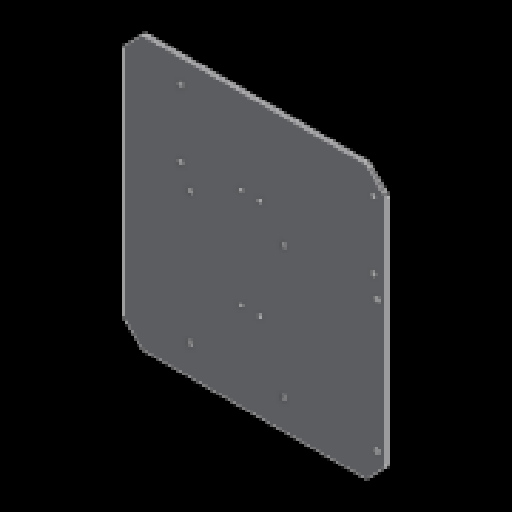
# Autodesk Inventor part: ChestTopPanel
Saved by Autodesk Inventor 2025.2 (Build 292293000, 293)
## iProperties
Created: 2025-10-05
Part Number: ChestTopPanel
Material: Generic
Document SubType Name: Sheet Metal
Designer: valer
Density: 1 g/cm^3
Sheet Metal Rule: Default
Appearance: Default
Author: valer
Autodesk Inventor part; units mm, degrees
ref_plane "YZ Plane" through (0, 0, 0) normal (1, 0, 0) x (0, 1, 0)
ref_plane "XZ Plane" through (0, 0, 0) normal (0, 1, 0) x (-1, 0, 0)
ref_plane "XY Plane" through (0, 0, 0) normal (0, 0, 1) x (1, 0, 0)
sketch "Base" plane through (0, 0, 0) normal (0, 0, 1) x (1, 0, 0)
  line L0 (370.5814, -184.5855) -> (20.5814, -184.5855)
  line L1 (20.5814, -184.5855) -> (20.5814, 180.4145)
  line L2 (20.5814, 180.4145) -> (370.5814, 180.4145)
  line L3 (370.5814, 180.4145) -> (370.5814, -184.5855)
  point P0 (0, 0)
  dimension "d1" = 365
  dimension "d3" = 350
  measures "d1" distance of L2.end L0.start
  measures "d3" distance of L0.start L0.end
extrude "Plate1" add sketch "Base" along normal blind 5
chamfer "BaseChamfersFeature" distance 25 angle 45 4 edges at (20.5814, 180.4145, 2.5) (370.5814, 180.4145, 2.5) (370.5814, -184.5855, 2.5) (20.5814, -184.5855, 2.5)
fillet "BaseFilletsFeature" radius 8 8 edges at (20.5814, 155.4145, 2.5) (45.5814, 180.4145, 2.5) (20.5814, -159.5855, 2.5) (45.5814, -184.5855, 2.5) (345.5814, 180.4145, 2.5) (370.5814, 155.4145, 2.5) (370.5814, -159.5855, 2.5) (345.5814, -184.5855, 2.5)
sketch "PowerSupplyBracketMountHoles" plane through (0, 0, 0) normal (0, 0, -1) x (-1, 0, 0)
  circle A0 centre (-360.5814, 31.4145) radius 3 projected
  circle A1 centre (-235.5814, 31.4145) radius 3 projected
  circle A2 centre (-110.5814, 31.4145) radius 3 projected
  circle A3 centre (-360.5814, -144.5855) radius 3 projected
  circle A4 centre (-235.5814, -144.5855) radius 3 projected
  circle A5 centre (-110.5814, -144.5855) radius 3 projected
  point P0 (0, 0)
extrude "PowerSupplyBracketMountHolesFeature" cut sketch "PowerSupplyBracketMountHoles" against normal blind 5
sketch "ChargerMountHoles" plane through (0, 0, 0) normal (0, 0, -1) x (-1, 0, 0)
  line L0 (-338.5814, 164.0145) -> (-338.5814, 43.4145) construction
  line L1 (-338.5814, 43.4145) -> (-358.8814, 43.4145) construction
  arc A0 (-364.5814, 49.1145) -> (-358.8814, 43.4145) centre (-358.8814, 49.1145) ccw construction
  line L2 (-364.5814, 49.1145) -> (-364.5814, 55.9145) construction
  line L3 (-364.5814, 55.9145) -> (-355.4314, 55.9145) construction
  arc A1 (-355.4314, 55.9145) -> (-355.4314, 61.6145) centre (-355.4314, 58.7645) ccw construction
  line L4 (-355.4314, 61.6145) -> (-364.5814, 61.6145) construction
  line L5 (-364.5814, 61.6145) -> (-364.5814, 145.8145) construction
  line L6 (-364.5814, 145.8145) -> (-355.4314, 145.8145) construction
  arc A2 (-355.4314, 145.8145) -> (-355.4314, 151.5145) centre (-355.4314, 148.6645) ccw construction
  line L7 (-355.4314, 151.5145) -> (-364.5814, 151.5145) construction
  line L8 (-364.5814, 151.5145) -> (-364.5814, 158.3145) construction
  arc A3 (-358.8814, 164.0145) -> (-364.5814, 158.3145) centre (-358.8814, 158.3145) ccw construction
  line L9 (-358.8814, 164.0145) -> (-338.5814, 164.0145) construction
  line L10 (-114.5814, 43.4145) -> (-114.5814, 164.0145) construction
  line L11 (-114.5814, 164.0145) -> (-94.2814, 164.0145) construction
  arc A4 (-88.5814, 158.3145) -> (-94.2814, 164.0145) centre (-94.2814, 158.3145) ccw construction
  line L12 (-88.5814, 158.3145) -> (-88.5814, 151.5145) construction
  line L13 (-88.5814, 151.5145) -> (-97.7314, 151.5145) construction
  arc A5 (-97.7314, 151.5145) -> (-97.7314, 145.8145) centre (-97.7314, 148.6645) ccw construction
  line L14 (-97.7314, 145.8145) -> (-88.5814, 145.8145) construction
  line L15 (-88.5814, 145.8145) -> (-88.5814, 61.6145) construction
  line L16 (-88.5814, 61.6145) -> (-97.7314, 61.6145) construction
  arc A6 (-97.7314, 61.6145) -> (-97.7314, 55.9145) centre (-97.7314, 58.7645) ccw construction
  line L17 (-97.7314, 55.9145) -> (-88.5814, 55.9145) construction
  line L18 (-88.5814, 55.9145) -> (-88.5814, 49.1145) construction
  arc A7 (-94.2814, 43.4145) -> (-88.5814, 49.1145) centre (-94.2814, 49.1145) ccw construction
  line L19 (-94.2814, 43.4145) -> (-114.5814, 43.4145) construction
  circle A8 centre (-97.7314, 58.7645) radius 2.5
  circle A9 centre (-97.7314, 148.6645) radius 2.5
  circle A10 centre (-355.4314, 58.7645) radius 2.5
  circle A11 centre (-355.4314, 148.6645) radius 2.5
  point P0 (0, 0)
  dimension "d14" = 5
  constraints: 4 centre point, 4 coincident, 3 equal radius
  measures "d14" diameter of A8
extrude "ChargerMountHolesFeature" cut sketch "ChargerMountHoles" against normal blind 5
sketch "USBHubMountHoles" plane through (0, 0, 0) normal (0, 0, -1) x (-1, 0, 0)
  circle A0 centre (-178.2994, 66.75) radius 2.25 construction
  circle A1 centre (-203.2994, 66.75) radius 2.25 construction
  circle A2 centre (-203.2994, -66.75) radius 2.25 construction
  circle A3 centre (-178.2994, -66.75) radius 2.25 construction
  circle A4 centre (-178.2994, 66.75) radius 1.75
  circle A5 centre (-203.2994, 66.75) radius 1.75
  circle A6 centre (-203.2994, -66.75) radius 1.75
  circle A7 centre (-178.2994, -66.75) radius 1.75
  point P0 (0, 0)
  dimension "d17" = 4.5
  dimension "d18" = 3.5
  constraints: 4 centre point, 4 coincident, 3 equal radius
  measures "d17" diameter of A0
  measures "d18" diameter of A4
extrude "USBHubMountHolesFeature" cut sketch "USBHubMountHoles" against normal blind 5
equation "\"d12\" = Thickness"
equation "\"d15\" = Thickness"
equation "\"d19\" = Thickness"
equation "\"d4\" = Thickness"
equation "\"BendRadius\" = Thickness"
equation "\"BendReliefWidth\" = Thickness"
equation "\"BendReliefDepth\" = 0.5 * Thickness"
equation "\"TransitionRadius\" = BendRadius"
equation "\"JacobiRadiusSize\" = BendRadius"
equation "\"GapSize\" = Thickness"
equation "\"Thickness\" = 5"
body "Solid1"
